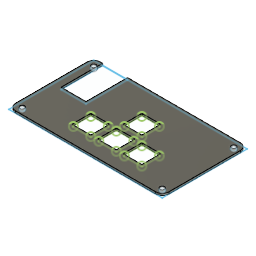
Hackpad_Full_Assembly (Autodesk Fusion 360 archive; units mm, degrees)
design "Top Case"
part number: 2026-03-30-22-45-58-601
Autodesk Fusion 360 part; units mm, degrees
sketch "Sketch1" plane through (0, 0, 0) normal (0, 0, 1) x (1, 0, 0)
  line L0 (57.075, 53.425) -> (70.075, 53.425)
  line L1 (57.075, 39.425) -> (70.075, 39.425)
  line L2 (56.575, 52.925) -> (56.575, 39.925)
  line L3 (70.575, 52.925) -> (70.575, 39.925)
  arc A0 (57.075, 53.425) -> (56.575, 52.925) centre (57.075, 52.925) ccw
  arc A1 (70.575, 52.925) -> (70.075, 53.425) centre (70.075, 52.925) ccw
  arc A2 (56.575, 39.925) -> (57.075, 39.425) centre (57.075, 39.925) ccw
  arc A3 (70.075, 39.425) -> (70.575, 39.925) centre (70.075, 39.925) ccw
  line L4 (38.025, 34.375) -> (51.025, 34.375)
  line L5 (38.025, 20.375) -> (51.025, 20.375)
  line L6 (37.525, 33.875) -> (37.525, 20.875)
  line L7 (51.525, 33.875) -> (51.525, 20.875)
  arc A4 (38.025, 34.375) -> (37.525, 33.875) centre (38.025, 33.875) ccw
  arc A5 (51.525, 33.875) -> (51.025, 34.375) centre (51.025, 33.875) ccw
  arc A6 (37.525, 20.875) -> (38.025, 20.375) centre (38.025, 20.875) ccw
  arc A7 (51.025, 20.375) -> (51.525, 20.875) centre (51.025, 20.875) ccw
  line L8 (57.075, 34.375) -> (70.075, 34.375)
  line L9 (57.075, 20.375) -> (70.075, 20.375)
  line L10 (56.575, 33.875) -> (56.575, 20.875)
  line L11 (70.575, 33.875) -> (70.575, 20.875)
  arc A8 (57.075, 34.375) -> (56.575, 33.875) centre (57.075, 33.875) ccw
  arc A9 (70.575, 33.875) -> (70.075, 34.375) centre (70.075, 33.875) ccw
  arc A10 (56.575, 20.875) -> (57.075, 20.375) centre (57.075, 20.875) ccw
  arc A11 (70.075, 20.375) -> (70.575, 20.875) centre (70.075, 20.875) ccw
  line L12 (76.125, 34.375) -> (89.125, 34.375)
  line L13 (76.125, 20.375) -> (89.125, 20.375)
  line L14 (75.625, 33.875) -> (75.625, 20.875)
  line L15 (89.625, 33.875) -> (89.625, 20.875)
  arc A12 (76.125, 34.375) -> (75.625, 33.875) centre (76.125, 33.875) ccw
  arc A13 (89.625, 33.875) -> (89.125, 34.375) centre (89.125, 33.875) ccw
  arc A14 (75.625, 20.875) -> (76.125, 20.375) centre (76.125, 20.875) ccw
  arc A15 (89.125, 20.375) -> (89.625, 20.875) centre (89.125, 20.875) ccw
  line L16 (117.3943, 71.2252) -> (2.8489, 71.2252)
  line L17 (2.8489, 71.2252) -> (2.8489, 7.8418)
  line L18 (2.8489, 7.8418) -> (117.3943, 7.8418)
  line L19 (117.3943, 7.8418) -> (117.3943, 71.2252)
  line L20 (9.5689, 71.2252) -> (28.0689, 71.2252)
  line L21 (28.0689, 71.2252) -> (28.0689, 40.2252)
  line L22 (28.0689, 40.2252) -> (9.5689, 40.2252)
  line L23 (9.5689, 40.2252) -> (9.5689, 71.2252)
  circle A16 centre (112.3943, 66.2252) radius 1.7
  circle A17 centre (112.3943, 12.8418) radius 1.7
  circle A18 centre (7.8489, 12.8418) radius 1.7
  circle A19 centre (7.8489, 66.2252) radius 1.7
  dimension "d1" = 114.5454
  dimension "d2" = 63.3834
  dimension "d3" = 37.513
  dimension "d5" = 18.5
  dimension "d6" = 31
  dimension "d7" = 6.72
  dimension "d8" = 3.4
  dimension "d9" = 5
  dimension "d10" = 5
  dimension "d11" = 3.4
  dimension "d12" = 5
  dimension "d13" = 5
  dimension "d14" = 3.4
  dimension "d15" = 5
  dimension "d16" = 5
  dimension "d17" = 3.4
  dimension "d18" = 5
  dimension "d19" = 5
  constraint horizontal L16
  constraint vertical L17
  constraint horizontal L18
  constraint vertical L19
  constraint horizontal L20
  constraint vertical L21
  constraint horizontal L22
  constraint vertical L23
  constraint coincident L16 L20.start
  measures "d1" distance of L16.start L16.end
  measures "d2" distance of L16.start L18.end
  measures "d3" distance of A6.centre L17.end
  measures "d5" distance of L20.start L20.end
  measures "d6" distance of L20.start L22.end
  measures "d7" distance of L16.end L20.start
  measures "d8" diameter of A16
  measures "d9" distance of L16 A16.centre
  measures "d10" distance of L19 A16.centre
  measures "d11" diameter of A17
  measures "d12" distance of L18 A17.centre
  measures "d13" distance of L19 A17.centre
  measures "d14" diameter of A18
  measures "d15" distance of L18 A18.centre
  measures "d16" distance of L17 A18.centre
  measures "d17" diameter of A19
  measures "d18" distance of L17 A19.centre
  measures "d19" distance of L16 A19.centre
extrude "Extrude1" add sketch "Sketch1" along normal blind 1.5 contours L16 L17 L18 L19 L21 L22 L23
fillet "Fillet1" radius 5 4 edges at (2.8489, 7.8418, 0.75) (2.8489, 71.2252, 0.75) (117.3943, 71.2252, 0.75) (117.3943, 7.8418, 0.75)

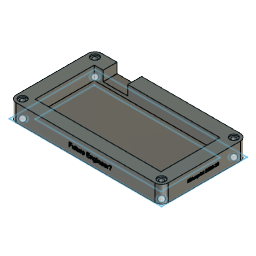
design "Hackpad1"
part number: 2026-03-18-16-25-58-676
Autodesk Fusion 360 part; units mm, degrees
sketch "Sketch1" plane through (0, 0, 0) normal (0, 0, 1) x (1, 0, 0)
  line L0 (-20, 50) -> (74.5454, 50)
  line L1 (74.5454, 50) -> (74.5454, 5.6166)
  line L2 (74.5454, 5.6166) -> (-20, 5.6166)
  line L3 (-20, 5.6166) -> (-20, 50)
  line L4 (-30, 60.5) -> (84.5454, 60.5)
  line L5 (84.5454, 60.5) -> (84.5454, -3.8834)
  line L6 (84.5454, -3.8834) -> (-30, -3.8834)
  line L7 (-30, -3.8834) -> (-30, 60.5)
  circle A0 centre (79.5454, 1.1166) radius 1.7
  circle A1 centre (-25, 1.1166) radius 1.7
  circle A2 centre (-25, 55.5) radius 1.7
  circle A3 centre (79.5454, 55.5) radius 1.7
  circle A4 centre (-25, 1.1166) radius 3
  circle A5 centre (-25, 55.5) radius 3
  circle A6 centre (79.5454, 55.5) radius 3
  circle A7 centre (79.5454, 1.1166) radius 3
  dimension "d1" = 94.5454
  dimension "d2" = 44.3834
  dimension "d3" = 114.5454
  dimension "d4" = 64.3834
  dimension "d5" = 9.5
  dimension "d7" = 3.4
  dimension "d8" = 5
  dimension "d9" = 5
  dimension "d10" = 3.4
  dimension "d11" = 5
  dimension "d12" = 5
  dimension "d13" = 3.4
  dimension "d14" = 5
  dimension "d15" = 5
  dimension "d16" = 3.4
  dimension "d17" = 5
  dimension "d18" = 5
  dimension "d19" = 6
  dimension "d20" = 6
  dimension "d21" = 6
  dimension "d22" = 6
  constraint horizontal L0
  constraint vertical L1
  constraint horizontal L2
  constraint vertical L3
  constraint horizontal L4
  constraint vertical L5
  constraint horizontal L6
  constraint vertical L7
  constraint concentric A1 A4
  constraint concentric A2 A5
  constraint concentric A3 A6
  constraint concentric A0 A7
  measures "d1" distance of L0.start L0.end
  measures "d2" distance of L0.start L2.end
  measures "d3" distance of L4.start L4.end
  measures "d4" distance of L4.start L6.end
  measures "d5" distance of L2 L6
  measures "d7" diameter of A0
  measures "d8" distance of L6 A0.centre
  measures "d9" distance of L5 A0.centre
  measures "d10" diameter of A1
  measures "d11" distance of L6 A1.centre
  measures "d12" distance of L7 A1.centre
  measures "d13" diameter of A2
  measures "d14" distance of L7 A2.centre
  measures "d15" distance of L4 A2.centre
  measures "d16" diameter of A3
  measures "d17" distance of L4 A3.centre
  measures "d18" distance of L5 A3.centre
  measures "d19" diameter of A4
  measures "d20" diameter of A5
  measures "d21" diameter of A6
  measures "d22" diameter of A7
extrude "Extrude1" add sketch "Sketch1" along normal blind 9 from surface at 3.1 contours A4 | A5 | A6 | A7 makes body 1 at (-22.0037, 0.9671, 9.1) makes body 2 at (80.3579, 4.0045, 9.1) makes body 3 at (-22.0037, 55.3505, 9.1) makes body 4 at (80.3579, 58.3879, 9.1)
extrude "Extrude2" add sketch "Sketch1" along normal blind 13 contours L4 L5 L6 L7 bodies 1 2 3 4
extrude "Extrude3" add sketch "Sketch1" along normal blind 3 contours L0 L1 L2 L3 bodies 1
sketch "Sketch2" plane through (0, 0, 13) normal (0, 0, 1) x (-1, 0, 0)
  line L0 (-74.5454, -5.6166) -> (20, -5.6166)
  line L1 (20, -5.6166) -> (20, -50)
  line L2 (20, -50) -> (-74.5454, -50)
  line L3 (-74.5454, -50) -> (-74.5454, -5.6166)
  circle A0 centre (25, -1.1166) radius 3
  circle A1 centre (25, -55.5) radius 3
  circle A2 centre (-79.5454, -1.1166) radius 3
  circle A3 centre (-79.5454, -55.5) radius 3
  line L4 (30, 3.8834) -> (-84.5454, 3.8834)
  line L5 (-84.5454, 3.8834) -> (-84.5454, -60.5)
  line L6 (-84.5454, -60.5) -> (30, -60.5)
  line L7 (30, -60.5) -> (30, 3.8834)
  line L8 (13.3043, -60.5) -> (-5.1957, -60.5)
  line L9 (-5.1957, -60.5) -> (-5.1957, -50.0173)
  line L10 (-5.1957, -50.0173) -> (13.3043, -50.0173)
  line L11 (13.3043, -50.0173) -> (13.3043, -60.5)
  line L12 (30, 3.8834) -> (30, -60.5)
  dimension "d30" = 18.5
  dimension "d41" = 16.6957
  constraint horizontal L8
  constraint vertical L9
  constraint horizontal L10
  constraint vertical L11
  constraint coincident L6 L8.start
  measures "d30" distance of L8.start L8.end
  measures "d41" distance of L11 L12
extrude "Extrude4" cut sketch "Sketch2" against normal blind 7.5 contours L6 L8 L9 L10 L11 bodies 1
fillet "Fillet1" radius 5 1 edges at (84.5454, 60.5, 6.5) on bodies 1
fillet "Fillet2" radius 5 1 edges at (-30, 60.5, 6.5) on bodies 1
fillet "Fillet3" radius 5 1 edges at (-30, -3.8834, 6.5) on bodies 1
fillet "Fillet4" radius 5 1 edges at (84.5454, -3.8834, 6.5) on bodies 1
extrude "Extrude5" cut sketch "Sketch2" against normal blind 7.5 contours L6 L8 L9 L10 L11 bodies 1
delete_face "DeleteFace1" 1 faces at (-0.9709, 50.0173, 8) on bodies 1
sketch "Sketch3" plane through (84.5454, 0, 0) normal (1, 0, 0) x (0, 1, 0)
  line L0 (1.1166, 13) -> (1.1166, 0)
  line L1 (1.1166, 0) -> (55.5, 0)
  line L2 (55.5, 0) -> (55.5, 13)
  line L3 (55.5, 13) -> (1.1166, 13)
  line L4 (13, 5) -> (42, 5) construction
  line L5 (42, 5) -> (42, 8) construction
  line L6 (42, 8) -> (13, 8) construction
  line L7 (13, 8) -> (13, 5) construction
  dimension "d44" = 2
  dimension "d45" = 0
  text T0 "#Blueprint 2025-26" font "Arial" height 2 align centre middle in box 29 x 3 at (13, 5) x (1, 0) y (0, 1) spacing 1 kerned
extrude "Extrude6" cut sketch "Sketch3" against normal blind 0.2 text T0 bodies 1
sketch "Sketch4" plane through (0, 0, 13) normal (0, 0, 1) x (-1, 0, 0)
  circle A0 centre (25, -1.1166) radius 3
  circle A1 centre (25, -55.5) radius 3
  line L0 (-5.1957, -60.5) -> (-5.1957, -50)
  line L1 (-5.1957, -50) -> (-74.5454, -50)
  line L2 (-74.5454, -50) -> (-74.5454, -5.6166)
  line L3 (-74.5454, -5.6166) -> (20, -5.6166)
  line L4 (20, -5.6166) -> (20, -50)
  line L5 (20, -50) -> (13.3043, -50)
  line L6 (13.3043, -50) -> (13.3043, -60.5)
  line L7 (13.3043, -60.5) -> (25, -60.5)
  arc A2 (25, -60.5) -> (30, -55.5) centre (25, -55.5) ccw
  line L8 (30, -55.5) -> (30, -1.1166)
  arc A3 (30, -1.1166) -> (25, 3.8834) centre (25, -1.1166) ccw
  line L9 (25, 3.8834) -> (-79.5454, 3.8834)
  arc A4 (-79.5454, 3.8834) -> (-84.5454, -1.1166) centre (-79.5454, -1.1166) ccw
  line L10 (-84.5454, -1.1166) -> (-84.5454, -55.5)
  arc A5 (-84.5454, -55.5) -> (-79.5454, -60.5) centre (-79.5454, -55.5) ccw
  line L11 (-79.5454, -60.5) -> (-5.1957, -60.5)
  circle A6 centre (-79.5454, -1.1166) radius 3
  circle A7 centre (-79.5454, -55.5) radius 3
sketch "Sketch5" plane through (-30, 0, 0) normal (-1, 0, 0) x (0, -1, 0)
  line L0 (-1.1166, 0) -> (-1.1166, 13)
  line L1 (-1.1166, 13) -> (-55.5, 13)
  line L2 (-55.5, 13) -> (-55.5, 0)
  line L3 (-55.5, 0) -> (-1.1166, 0)
  line L4 (-44, 4) -> (-13, 4) construction
  line L5 (-13, 4) -> (-13, 8) construction
  line L6 (-13, 8) -> (-44, 8) construction
  line L7 (-44, 8) -> (-44, 4) construction
  dimension "d48" = 3
  dimension "d49" = 0
  text T0 "HACKPAD v1.0" font "Arial" height 3 align centre middle in box 31 x 4 at (-44, 4) x (1, 0) y (0, 1) spacing 1 kerned
extrude "Extrude7" add sketch "Sketch5" along normal blind 0.2 text T0 bodies 1
sketch "Sketch6" plane through (0, -3.8834, 0) normal (0, -1, 0) x (1, 0, 0)
  line L0 (79.5454, 0) -> (79.5454, 13)
  line L1 (79.5454, 13) -> (-25, 13)
  line L2 (-25, 13) -> (-25, 0)
  line L3 (-25, 0) -> (79.5454, 0)
  line L4 (1, 4) -> (61, 4) construction
  line L5 (61, 4) -> (61, 8) construction
  line L6 (61, 8) -> (1, 8) construction
  line L7 (1, 8) -> (1, 4) construction
  dimension "d52" = 3
  text T0 "Future Engineer?" font "Arial" height 3 align centre middle in box 60 x 4 at (1, 4) x (1, 0) y (0, 1) spacing 1 kerned
extrude "Extrude8" add sketch "Sketch6" along normal blind 0.2 text T0 bodies 1
equation "d45 = '#Blueprint 2025-26'"
equation "d49 = 'HACKPAD v1.0'"
equation "d53 = 'Future Engineer?'"
